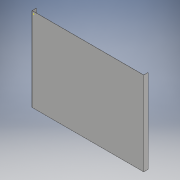
# Autodesk Inventor part: Полка
Saved by Autodesk Inventor 2017 (Build 210142000, 142)
## iProperties
Part Number: Полка
Material: Типовые
Document SubType Name: Modeling
Designer: CAD_Admin
Density: 1 g/cm^3
Appearance: По умолчанию
Author: CAD_Admin
Autodesk Inventor part; units mm, degrees
ref_plane "YZ Plane" through (0, 0, 0) normal (1, 0, 0) x (0, 1, 0)
ref_plane "XZ Plane" through (0, 0, 0) normal (0, 1, 0) x (-1, 0, 0)
ref_plane "XY Plane" through (0, 0, 0) normal (0, 0, 1) x (1, 0, 0)
sketch "Эскиз1" plane through (0, 0, 0) normal (0, 1, 0) x (-1, 0, 0)
  line L0 (13.83, 15.6551) -> (-786.17, 15.6551)
  line L1 (-786.17, 15.6551) -> (-786.17, -584.3449)
  line L2 (-786.17, -584.3449) -> (13.83, -584.3449)
  line L3 (13.83, -584.3449) -> (13.83, 15.6551)
  point P0 (0, 0)
  dimension "d0" = 800
  dimension "d1" = 600
  constraints: 8 end point, 2 parallel, 1 horizontal, 1 perpendicular
  measures "d0" distance of L2.end L1.end
  measures "d1" distance of L1.end L0.end
extrude "Выдавливание1" add sketch "Эскиз1" along normal blind 1
sketch "Эскиз2" plane through (0, 1, 0) normal (0, 1, 0) x (1, 0, 0)
  point P0 (0, 0)
sketch "Эскиз3" plane through (0, 1, 0) normal (0, 1, 0) x (1, 0, 0)
  line L0 (-13.83, 584.3449) -> (-13.83, -15.6551) projected
  line L1 (-13.83, -15.6551) -> (-12.83, -15.6551)
  line L2 (-12.83, -15.6551) -> (-12.83, 584.3449)
  line L3 (-12.83, 584.3449) -> (-13.83, 584.3449)
  line L4 (-13.83, 584.3449) -> (-13.83, -15.6551)
  line L5 (-13.83, -15.6551) -> (786.17, -15.6551) projected
  line L6 (786.17, -15.6551) -> (785.17, -15.6551)
  line L7 (785.17, -15.6551) -> (785.17, 584.3449)
  line L8 (785.17, 584.3449) -> (786.17, 584.3449)
  line L9 (786.17, 584.3449) -> (786.17, -15.6551)
  point P0 (0, 0)
  dimension "d4" = 1
  dimension "d5" = 600
  dimension "d6" = 1
  dimension "d7" = 600
  constraints: 16 end point, 4 parallel, 2 horizontal, 2 perpendicular
  measures "d4" distance of L3.end L2.end
  measures "d5" distance of L2.end L1.end
  measures "d6" distance of L7.end L8.end
  measures "d7" distance of L6.end L7.end
extrude "Выдавливание2" add sketch "Эскиз3" along normal blind 30 contours L3 L2 L1 L0
sketch "Эскиз4" plane through (0, 1, 0) normal (0, 1, 0) x (1, 0, 0)
  line L0 (786.17, -15.6551) -> (785.17, -15.6551)
  line L1 (785.17, -15.6551) -> (785.17, 584.3449)
  line L2 (785.17, 584.3449) -> (786.17, 584.3449)
  line L3 (786.17, 584.3449) -> (786.17, -15.6551)
  point P0 (0, 0)
  dimension "d10" = 1
  dimension "d11" = 600
  constraints: 8 end point, 2 parallel, 1 horizontal, 1 perpendicular
  measures "d10" distance of L1.end L2.end
  measures "d11" distance of L0.end L1.end
extrude "Выдавливание3" add sketch "Эскиз4" along normal blind 30
